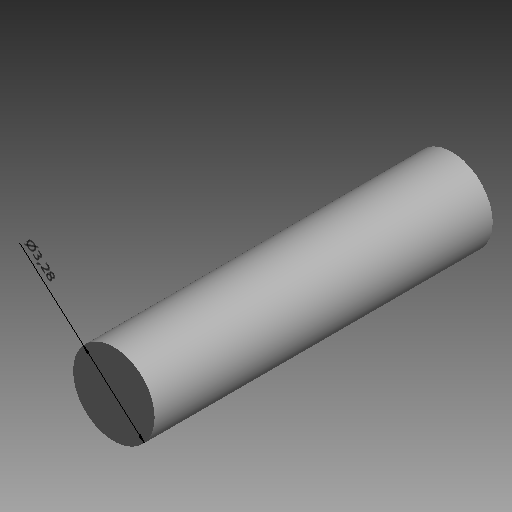
# Autodesk Inventor part: 06B - 1 RP- Pin 2
Saved by Autodesk Inventor 2019 (Build 230136000, 136)
## iProperties
Category: PARTsolutions
Company: KANA
Part Number: 06B - 1 RP- Pin 2
Material: 一般
Catalog Web Link: www.cadenas.de
Description: Standard Chain Pin 2-
Vendor: KANA
Document SubType Name: Modeling
Designer: partserver
Manufacturer: KANA
Mass: 0.114915 g
Surface Area: 1.57039 cm^2
Volume: 0.114915 cm^3
Density: 1 g/cm^3
Appearance: PSOLRGB-192-192-192
PSOL_IDENT_0: {$CADENAS_DATA\23d-libs\kana\roller_chain\standard_chain\standard_chain_body2_a.prj},187 {VTYP=3D},{
PSOL_IDENT_1: NB=06B - 1 RP- Pin 2},{LINA=06B - 1 RP},{NN=Standard Chain Pin 2},{DATE=04.07.2018 01:10:23},{GEOMDA
PSOL_IDENT_2: TE=12.09.2016 11:10:15},{VERSION=},{LINEID=10},{WBVAR=NOL},{WBNUMERIC=NOL}  {NB=06B - 1 RP- Pin 2},{
PSOL_IDENT_3: LINA=06B - 1 RP},{KT=DUMMY},{CNO=06B},{PT=RP},{NOL=1},{NOLX=1},{P=9.525},{R=6.350},{W=5.720},{T=1.00
PSOL_IDENT_4: 0},{H=8.100},{D=3.280},{L=13.6},{C=10.24},{L1=6.1},{L2=7.5},{C11=0},{VER=2}
NB: 06B - 1 RP- Pin 2
NN: Standard Chain Pin 2
NBSYN: $CNO. - $NOL. $PT.- Pin 2
LINA: 06B - 1 RP
CATALOG: KANA
CNO: 06B
PT: RP
NOL: 1
P: 9.525
R: 6.35
W: 5.72
T: 1
H: 8.1
D: 3.28
VER: 2
SUPPLIER: KANA
ARTICLENO: 06B - 1 RP- Pin 2
BOMINFO: 06B - 1 RP
CREATOR: CADENAS GmbH
Title: 06B - 1 RP
Author: Cadenas PARTsolutions
Autodesk Inventor part; units mm, degrees
sketch "Sketch_1" plane through (0, 0, 0) normal (0, 0, 1) x (1, 0, 0)
  line L0 (0, -7.5) -> (0, 6.1)
  line L1 (0, 6.1) -> (1.64, 6.1)
  line L2 (1.64, 6.1) -> (1.64, -7.5)
  line L3 (1.64, -7.5) -> (0, -7.5)
  line L4 (0, -7.5) -> (0, 6.1)
  constraints: 10 end point
revolve "Revolution1" add sketch "Sketch_1" angle 360 about axis through (0, -7.5, 0) along (0, -1, 0)
ref_plane "Body2_1_XY" through (0, 0, 0) normal (0, 1, 0) x (1, 0, 0)
ref_plane "Body2_1_YZ" through (0, 0, 0) normal (1, 0, 0) x (0, 0, -1)
ref_plane "Body2_1_ZX" through (0, 0, 0) normal (0, 0, -1) x (0, 1, 0)
body "Solid1"
